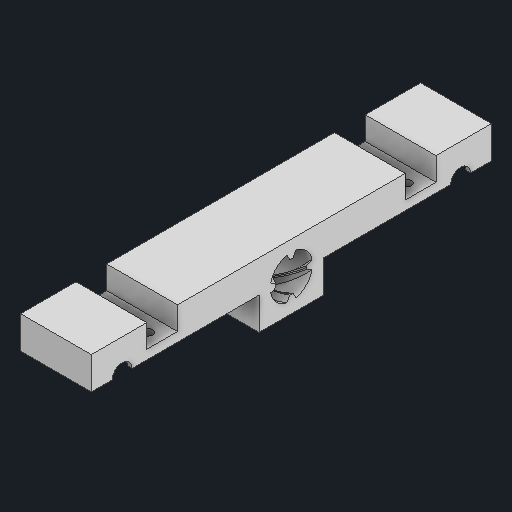
# Autodesk Inventor part: screw_slider
Saved by Autodesk Inventor 2025 (Build 290162010, 162A)
## iProperties
Created: 2024-06-23
Part Number: screw_slider
Material: Generic
Document SubType Name: Modeling
Designer: mihir
Density: 1 g/cm^3
Appearance: Default
Author: mihir
Autodesk Inventor part; units mm, degrees
ref_plane "YZ Plane" through (0, 0, 0) normal (1, 0, 0) x (0, 1, 0)
ref_plane "XZ Plane" through (0, 0, 0) normal (0, 1, 0) x (-1, 0, 0)
sketch "Sketch1" plane through (0, 0, 0) normal (0, 1, 0) x (-1, 0, 0)
  line L0 (0, 0) -> (23, 0)
  line L1 (23, 0) -> (23, -130)
  line L2 (23, -130) -> (0, -130)
  line L3 (0, -130) -> (0, 0)
  dimension "d0" = 130
  dimension "d1" = 23
  constraints: 8 end point, 2 parallel, 1 horizontal, 1 perpendicular
  measures "d0" distance of L2.end L0.start
  measures "d1" distance of L0.start L0.end
extrude "Extrusion1" add sketch "Sketch1" along normal blind 10.5
sketch "Sketch2" plane through (0, 0, 0) normal (0, -1, 0) x (1, 0, 0)
  line L0 (-1.5, -4) -> (-21.5, -4)
  line L1 (-21.5, -4) -> (-21.5, -10)
  line L2 (-21.5, -10) -> (-1.5, -10)
  line L3 (-1.5, -10) -> (-1.5, -4)
  line L4 (-23, 0) -> (0, 0) projected
  line L5 (0, 0) -> (0, -130) projected
  line L6 (0, 0) -> (0, -130) construction
  line L7 (0, -40) -> (-23, -40) construction
  line L8 (-23, -130) -> (-23, 0) construction
  dimension "d4" = 6
  dimension "d5" = 20
  dimension "d6" = 4
  dimension "d7" = 1.5
  dimension "d8" = 40
  constraints: 10 end point, 2 horizontal, 2 parallel, 2 point on line, 1 perpendicular
  measures "d4" distance of L2.end L0.start
  measures "d5" distance of L0.start L0.end
  measures "d6" distance between parallel lines of L4 L0
  measures "d7" distance between parallel lines of L5 L3
  measures "d8" distance between parallel lines of L4 L7
revolve "Revolution1" cut sketch "Sketch2" angle 360 about axis through (-21.5, 0, -10) along (1, 0, 0)
sketch "Sketch3" plane through (0, 0, 0) normal (0, -1, 0) x (1, 0, 0)
  line L0 (0, 0) -> (0, -130) construction
  line L1 (0, -40) -> (-23, -40) construction
  line L2 (-23, -130) -> (-23, 0) construction
  line L3 (-23, 0) -> (0, 0) construction
  line L4 (-4.5, -23) -> (-18.5, -23) construction
  line L5 (-11.5, -23) -> (-11.5, -40) construction
  dimension "d10" = 40
  dimension "d12" = 14
  dimension "d46" = 23
  constraints: 6 end point, 2 horizontal, 2 midpoint, 2 point on line, 1 vertical
  measures "d10" distance between parallel lines of L3 L1
  measures "d12" distance of L4.end L4.start
  measures "d46" distance from line of L3 L4.start
hole "Hole1" at (-4.5, 0, -23) at (-18.5, 0, -23) direction (0, 1, 0) diameter 3 depth 10.5
sketch "Sketch4" plane through (0, 10.5, 0) normal (0, 1, 0) x (1, 0, 0)
  line L0 (-23, 130) -> (-23, 0) projected
  line L1 (0, 0) -> (0, 130) projected
  line L2 (-23, 18) -> (0, 18)
  line L3 (0, 18) -> (0, 28)
  line L4 (0, 28) -> (-23, 28)
  line L5 (-23, 28) -> (-23, 18)
  circle A0 centre (-18.5, 23) radius 1.5 construction
  circle A1 centre (-4.5, 23) radius 1.5 construction
  line L6 (-18.5, 23) -> (-4.5, 23) construction
  line L7 (-23, 0) -> (0, 0) construction
  line L8 (-11.5, 0) -> (-11.5, 18) construction
  point P0 (-23, 28)
  point P1 (0, 18)
  dimension "d20" = 10
  dimension "d45" = 18
  constraints: 12 end point, 2 horizontal, 2 midpoint, 2 parallel, 2 point on line, 1 perpendicular
  measures "d20" distance between parallel lines of L2 L4
  measures "d45" distance of L8.start L8.end
extrude "Extrusion2" cut sketch "Sketch4" against normal blind 7.5
ref_plane "Work Plane1" through (-23, 0, -65) normal (0, 0, 1) x (1, 0, 0)
mirror "Mirror1" about plane through (-23, 0, -65) normal (0, 0, 1) of "Revolution1", "Hole1", "Extrusion2"
sketch "Sketch5" plane through (0, 0, 0) normal (1, 0, 0) x (0, 0, -1)
  circle A0 centre (65, 0) radius 6.875
  line L0 (0, 0) -> (130, 0) projected
  line L1 (28, 10.5) -> (102, 10.5) projected
  line L2 (54.5, -10.5) -> (75.5, -10.5)
  line L3 (75.5, -10.5) -> (75.5, 10.5)
  line L4 (75.5, 10.5) -> (54.5, 10.5)
  line L5 (54.5, 10.5) -> (54.5, -10.5)
  line L6 (54.5, -10.5) -> (75.5, 10.5) construction
  line L7 (75.5, -10.5) -> (54.5, 10.5) construction
  point P0 (75.5, 0)
  point P1 (71.875, 0)
  point P2 (58.125, 0)
  point P3 (54.5, 0)
  dimension "d23" = 13.75
  constraints: 12 end point, 3 midpoint, 2 parallel, 2 perpendicular, 1 centre point, 1 coincident, 1 horizontal, 1 point on line
  measures "d23" diameter of A0
extrude "Extrusion3" add sketch "Sketch5" against normal up to surface (23 mm away) contours L0 L3 L2 L5 A0
sketch "Sketch6" plane through (0, 0, -130) normal (1, 0, 0) x (0, 0, -1)
  line L0 (-58.125, 0) -> (-71.875, 0) projected
  arc A0 (-58.125, 0) -> (-71.875, 0) centre (-65, 0) ccw
  line L1 (-71.875, 0) -> (-58.125, 0)
  point P0 (-130, 0)
  constraints: 2 end point, 2 point on circle, 1 centre point, 1 collinear, 1 midpoint
extrude "Extrusion4" cut sketch "Sketch6" against normal up to surface (23 mm away)
sketch "Sketch7" plane through (0, 0, -130) normal (1, 0, 0) x (0, 0, -1)
  circle A0 centre (-65, 0) radius 6.875 construction
  circle A1 centre (-65, 0) radius 5 construction
  line L0 (-70, 0) -> (-70, 0.5)
  line L1 (-70, 0.5) -> (-71.875, 1.5825)
  line L2 (-71.875, 1.5825) -> (-71.875, 0)
  line L3 (-71.875, 0) -> (-70, 0)
  line L4 (-70, 0) -> (-70, -0.5)
  line L5 (-70, -0.5) -> (-71.875, -1.5825)
  line L6 (-71.875, -1.5825) -> (-71.875, 0)
  point P0 (-130, 0)
  dimension "d28" = 10
  dimension "d29" = 120
  dimension "d30" = 0.5
  constraints: 14 end point, 3 vertical, 2 horizontal alignment, 2 symmetric about line, 1 coincident, 1 horizontal, 3 other
  measures "d30" distance of L0.start L0.end
coil "Coil1" sketch "Sketch7" operation add axis through (0, 0, -65) along (-1, 0, 0) pitch 40 turns 0.575 hand right
pattern_circular "Circular Pattern1" count 4 over 360 about axis through (0, 0, -65) along (-1, 0, 0) of "Coil1"
sketch "Sketch8" plane through (0, 0, -130) normal (1, 0, 0) x (0, 0, -1)
  arc A0 (-114, 0) -> (-126, 0) centre (-120, 0) ccw projected
  arc A1 (-4, 0) -> (-16, 0) centre (-10, 0) ccw projected
  line L0 (-130, 0) -> (-75.5, 0) projected
  arc A2 (-116.75, 0) -> (-123.25, 0) centre (-120, 0) ccw
  line L1 (-123.25, 0) -> (-116.75, 0)
  point P0 (-123.25, 0)
  dimension "d42" = 3.25
  constraints: 2 end point, 2 point on circle, 1 centre point, 1 coincident, 1 collinear, 1 point on line
  measures "d42" radius of A2
extrude "Extrusion5" cut sketch "Sketch8" against normal up to surface (23 mm away) contours L0 A2
mirror "Mirror2" about plane through (-23, 0, -65) normal (0, 0, 1) of "Extrusion5"
equation "\"d0\" = table_bed_width"
equation "\"d1\" = table_bed_peg_width"
equation "\"d4\" = 0.5 * bearing_diameter"
equation "\"d5\" = bearing_length"
equation "\"d7\" = 0.5 * table_bed_peg_width - 0.5 * bearing_length"
equation "\"d8\" = table_bed_peg_length"
equation "\"d10\" = table_bed_peg_length"
equation "\"d12\" = screw_x"
equation "\"d46\" = screw_y"
equation "\"d13\" = screw_diameter"
equation "\"d20\" = cutout_width"
equation "\"d23\" = lead_screw_outer_diameter"
equation "\"d28\" = lead_screw_diameter"
equation "\"d29\" = screw_profile_angle"
equation "\"d30\" = 0.5 * screw_profile_width"
equation "\"d31\" = screw_pitch"
equation "\"d42\" = 0.5 * rod_free_tolerance + 0.5 * rod_diameter"
equation "\"table_bed_width\" = 130"
equation "\"table_bed_peg_width\" = 23"
equation "\"screw_slider_thickness\" = 10.5"
equation "\"bearing_length\" = 20"
equation "\"bearing_diameter\" = 12"
equation "\"table_bed_peg_length\" = 40"
equation "\"screw_y\" = 23"
equation "\"screw_x\" = 14"
equation "\"screw_diameter\" = 3"
equation "\"cutout_width\" = 10"
equation "\"lead_screw_outer_diameter\" = 13.75"
equation "\"screw_profile_width\" = 1"
equation "\"screw_profile_angle\" = 120deg"
equation "\"screw_pitch\" = 40"
equation "\"rod_diameter\" = 6"
equation "\"rod_free_tolerance\" = 0.5"
equation "\"lead_screw_diameter\" = 10"
body "Solid1"
